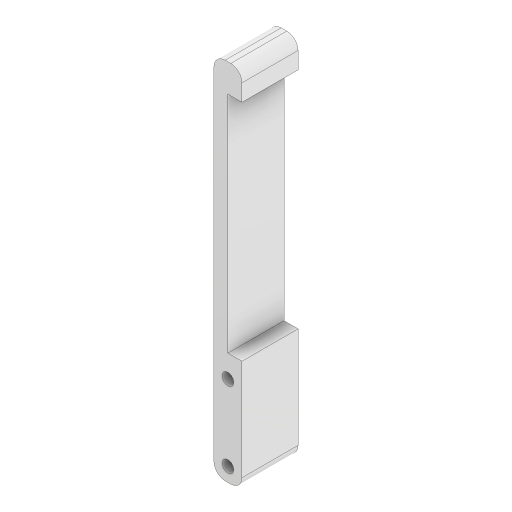
# Autodesk Inventor part: finger1
Saved by Autodesk Inventor 2024.3 (Build 283343000, 343)
## iProperties
Created: 2024-10-15
Part Number: finger1
Material: アセタール樹脂、白
Document SubType Name: Modeling
Designer: haya
Density: 1.425 g/cm^3
Appearance: 滑らか - 白
Mass: 20.1939 g
Surface Area: 64.0756 cm^2
Volume: 14.1711 cm^3
Author: haya
Autodesk Inventor part; units mm, degrees
ref_plane "YZ Plane" through (0, 0, 0) normal (1, 0, 0) x (0, 1, 0)
ref_plane "XZ Plane" through (0, 0, 0) normal (0, 1, 0) x (-1, 0, 0)
ref_plane "XY Plane" through (0, 0, 0) normal (0, 0, 1) x (1, 0, 0)
sketch "スケッチ1" plane through (0, 0, 0) normal (0, 0, 1) x (1, 0, 0)
  line L0 (0, 0) -> (10, 0)
  line L1 (10, 0) -> (10, 130)
  line L2 (10, 130) -> (0, 130)
  line L3 (0, 130) -> (0, 0)
  dimension "d0" = 10
  dimension "d1" = 130
  constraints: 8 end point, 2 parallel, 1 horizontal, 1 perpendicular
  measures "d0" distance of L0.start L0.end
  measures "d1" distance of L2.end L0.start
extrude "押し出し1" add sketch "スケッチ1" along normal blind 20
sketch "スケッチ2" plane through (0, 0, 20) normal (0, 0, 1) x (1, 0, 0)
  line L0 (10, 130) -> (0, 130) projected
  line L1 (5, 130) -> (5, 0) construction
  line L2 (0, 0) -> (10, 0) projected
  point P0 (5, 5)
  point P1 (5, 32)
  dimension "d4" = 27
  dimension "d5" = 5
  constraints: 2 end point, 2 midpoint, 2 point on line
  measures "d4" distance of point (5, 32) point (5, 5)
  measures "d5" distance from line of point (5, 5) L2
hole "穴1" at (5, 5, 20) at (5, 32, 20) direction (0, 0, -1) diameter 4.2 depth 20
sketch "スケッチ3" plane through (10, 0, 0) normal (1, 0, 0) x (0, 0, -1)
  line L0 (-20, 0) -> (-20, 130) projected
  line L1 (0, 0) -> (0, 130) projected
  line L2 (-20, 120) -> (0, 120)
  line L3 (0, 120) -> (0, 40)
  line L4 (0, 40) -> (-20, 40)
  line L5 (-20, 40) -> (-20, 120)
  line L6 (0, 130) -> (-20, 130) projected
  point P0 (-10, 120)
  point P1 (-20, 40)
  point P2 (0, 120)
  dimension "d13" = 10
  dimension "d14" = 80
  constraints: 8 end point, 2 parallel, 2 point on line, 1 horizontal, 1 midpoint, 1 perpendicular
  measures "d13" distance from line of point (-10, 120) L6
  measures "d14" distance between parallel lines of L4 L2
extrude "押し出し2" cut sketch "スケッチ3" against normal blind 5 contours L0 L2 L1 L4
fillet "フィレット1" radius 4 4 edges at (10, 0, 10) (0, 0, 10) (10, 130, 10) (0, 130, 10)
